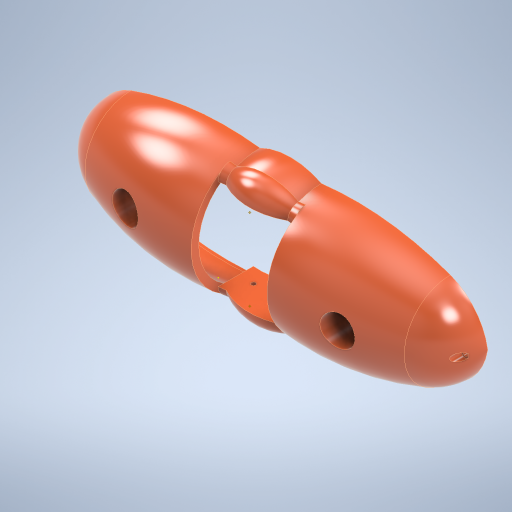
# Autodesk Inventor part: przód
Saved by Autodesk Inventor 2024 (Build 280153000, 153)
## iProperties
Created: 2025-05-21
Part Number: przód
Material: Tworzywo sztuczne PET
Document SubType Name: Modeling
Designer: Paweł
Density: 1.541 g/cm^3
Appearance: Gładki — jasnopomarańczowy
Mass: 215.204 g
Surface Area: 613.74 cm^2
Volume: 139.652 cm^3
Author: Paweł
Autodesk Inventor part; units mm, degrees
ref_plane "YZ Plane" through (0, 0, 0) normal (1, 0, 0) x (0, 1, 0)
sketch "Szkic1" plane through (0, 0, 0) normal (0, 0, 1) x (1, 0, 0)
  line L0 (19.3649, 0) -> (-19.3649, 0)
  line L1 (-19.3649, 0) -> (-103.6215, 0)
  line L2 (-103.6215, 0) -> (-125, 0)
  line L3 (-125, 0) -> (-103.6215, 0)
  line L4 (-103.6215, 0) -> (-19.3649, 0)
  line L5 (-19.3649, 0) -> (19.3649, 0)
  line L6 (19.3649, 0) -> (103.6215, 0)
  line L7 (103.6215, 0) -> (125, 0)
  line L8 (125, 0) -> (103.6215, 0)
  line L9 (103.6215, 0) -> (19.3649, 0)
  line L10 (45, 0) -> (-45, 0)
  line L11 (45, 0) -> (105.3748, 0)
  line L12 (105.3748, 0) -> (130.0712, 0)
  line L13 (130.0712, 0) -> (105.3748, 0)
  line L14 (105.3748, 0) -> (-20.2973, 0)
  line L15 (-20.2973, 0) -> (-105.3748, 0)
  line L16 (-105.3748, 0) -> (-105.3748, 0)
  line L17 (-105.3748, 0) -> (-130.0712, 0)
  line L18 (-130.0712, 0) -> (-105.3748, 0)
  line L19 (-105.3748, 0) -> (-45, 0)
  arc A0 (119.2902, -19.1594) -> (125, 0) centre (90, 0) ccw
  arc A1 (19.3649, -35) -> (103.6215, -25.7743) centre (42.8262, 140.0954) ccw
  arc A2 (103.6215, -25.7743) -> (125, 0) centre (91.4189, 6.1005) ccw
  arc A3 (20.2973, -40.1624) -> (105.3748, -30.457) centre (42.8262, 140.0954) ccw
  arc A4 (105.3748, -30.457) -> (130.0712, 0) centre (91.4189, 6.1005) ccw
  arc A5 (-125, 0) -> (-103.6215, -25.7743) centre (-91.4189, 6.1005) ccw
  arc A6 (-130.0712, 0) -> (-105.3748, -30.457) centre (-91.4189, 6.1005) ccw
  arc A7 (-98.4086, -33.9749) -> (-78.2644, -32.9739) centre (-90, 0) ccw
  arc A8 (-103.6215, -25.7743) -> (-19.3649, -35) centre (-42.8262, 140.0954) ccw
  arc A9 (-19.3649, -35) -> (19.3649, -35) centre (0, 0) ccw
  arc A10 (-20.2973, -40.1624) -> (20.2973, -40.1624) centre (0, 0) ccw
  arc A11 (-105.3748, -30.457) -> (-20.2973, -40.1624) centre (-42.8262, 140.0954) ccw
  line L20 (-105.3748, 0) -> (-20.2973, 0)
  line L21 (19.3649, 0) -> (-19.3649, 0)
  line L22 (130.0712, 0) -> (-130.0712, 0)
  point P0 (0, 0)
  point P1 (-119.2902, -19.1594)
  point P2 (-125, 0)
  point P3 (125, 0)
  dimension "d0" = 70
  dimension "d1" = 70
  dimension "d2" = 250
  dimension "d3" = 90
  constraints: 46 end point, 25 point on circle, 12 centre point, 2 horizontal alignment, 1 coincident, 1 horizontal, 4 other
  measures "d0" diameter of A0
  measures "d1" diameter of A7
  measures "d3" distance of point (0, 0) A7.centre
revolve "Obrót1" add sketch "Szkic1" angle 180 about axis through (130.0712, 0, 0) along (-1, 0, 0) contours L12 A4 A3 A10 A11 A7 A8 A9 A1 A2 | A5 A8 A7 A11 A6 L17
sketch "Szkic2" plane through (0, 0, 0) normal (0, 1, 0) x (-1, 0, 0)
  line L0 (-25, 45) -> (25, 45)
  line L1 (25, 45) -> (25, 15)
  line L2 (25, 15) -> (-25, 15)
  line L3 (-25, 15) -> (-25, 45)
  line L4 (-20.2973, 0) -> (20.2973, 0) projected
  arc A0 (105.3748, 30.457) -> (20.2973, 40.1624) centre (42.8262, -140.0954) ccw projected
  arc A1 (20.2973, 40.1624) -> (-20.2973, 40.1624) centre (0, 0) ccw projected
  point P0 (0, 0)
  point P1 (0, 45)
  point P2 (0, 0)
  point P3 (0, 45)
  dimension "d5" = 50
  dimension "d6" = 30
  constraints: 8 end point, 3 perpendicular, 2 midpoint, 1 coincident, 1 horizontal, 1 point on circle, 1 vertical alignment
  measures "d5" distance of L0.start L0.end
  measures "d6" distance of L0.end L1.end
extrude "Wyciągnięcie proste1" cut sketch "Szkic2" along normal mid plane 91
sketch "Szkic3" plane through (25, 0, 0) normal (-1, 0, 0) x (0, 0, 1)
  point P0 (0, 0)
sketch "Szkic11" plane through (0, 0, 15) normal (0, 0, 1) x (1, 0, 0)
  spline S0 degree 4 poles (25, -37.8222) (23.8224, -37.6973) (22.646, -37.5613) (21.4709, -37.4143) (20.2973, -37.2561) knots 0 0 0 0 0 1 1 1 1 1 projected
  line L0 (25, -32.3552) -> (25, -37.8222) projected
  spline S1 degree 7 poles (19.3649, -31.6228) (19.9801, -31.714) (20.5958, -31.8024) (21.2118, -31.888) (21.8282, -31.9707) (22.445, -32.0506) (23.0621, -32.1277) (23.8682, -32.2247) (24.0567, -32.2471) (24.2453, -32.2692) (24.4339, -32.2911) (24.6226, -32.3127) (24.8113, -32.3341) (25, -32.3552) knots 0 0 0 0 0 0 0 0 0.766096 0.766096 0.766096 0.766096 0.766096 0.766096 1 1 1 1 1 1 1 1 projected
  arc A0 (-19.3649, -31.6228) -> (19.3649, -31.6228) centre (0, 0) ccw projected
  spline S2 degree 4 poles (-25, -32.3552) (-23.5881, -32.1973) (-22.1781, -32.0227) (-20.7702, -31.8312) (-19.3649, -31.6228) knots 0 0 0 0 0 1 1 1 1 1 projected
  line L1 (-25, -37.8222) -> (-25, -32.3552) projected
  spline S3 degree 4 poles (-20.2973, -37.2561) (-21.4709, -37.4143) (-22.646, -37.5613) (-23.8224, -37.6973) (-25, -37.8222) knots 0 0 0 0 0 1 1 1 1 1 projected
  arc A1 (-20.2973, -37.2561) -> (20.2973, -37.2561) centre (0, 0) ccw projected
  line L2 (20, -30) -> (-20, -30) projected
  line L3 (-25, -30) -> (-20, -30) projected
  line L4 (-25, -32.3552) -> (-25, -30)
  line L5 (25, -32.3552) -> (25, -30)
  line L6 (25, -30) -> (20, -30)
  point P0 (0, 0)
  constraints: 6 end point, 2 perpendicular, 1 point on line, 4 other
revolve "Obrót2" add sketch "Szkic11" angle 105 about axis through (20, -30, 15) along (-1, 0, 0) contours S0 A1 S3 L1 S2 A0 S1 L0
sketch "Szkic12" plane through (0, 0, 15) normal (0, 0, 1) x (1, 0, 0)
  spline S0 degree 4 poles (20.2973, 37.2561) (21.4709, 37.4143) (22.646, 37.5613) (23.8224, 37.6973) (25, 37.8222) knots 0 0 0 0 0 1 1 1 1 1 projected
  arc A0 (20.2973, 37.2561) -> (-20.2973, 37.2561) centre (0, 0) ccw projected
  spline S1 degree 4 poles (-25, 37.8222) (-23.8224, 37.6973) (-22.646, 37.5613) (-21.4709, 37.4143) (-20.2973, 37.2561) knots 0 0 0 0 0 1 1 1 1 1 projected
  line L0 (-25, 32.3552) -> (-25, 37.8222) projected
  spline S2 degree 4 poles (-19.3649, 31.6228) (-20.7702, 31.8312) (-22.1781, 32.0227) (-23.5881, 32.1973) (-25, 32.3552) knots 0 0 0 0 0 1 1 1 1 1 projected
  arc A1 (19.3649, 31.6228) -> (-19.3649, 31.6228) centre (0, 0) ccw projected
  spline S3 degree 7 poles (25, 32.3552) (24.8113, 32.3341) (24.6226, 32.3127) (24.4339, 32.2911) (24.2453, 32.2692) (24.0567, 32.2471) (23.8682, 32.2247) (23.0621, 32.1277) (22.445, 32.0506) (21.8282, 31.9707) (21.2118, 31.888) (20.5958, 31.8024) (19.9801, 31.714) (19.3649, 31.6228) knots 0 0 0 0 0 0 0 0 0.233904 0.233904 0.233904 0.233904 0.233904 0.233904 1 1 1 1 1 1 1 1 projected
  line L1 (25, 37.8222) -> (25, 32.3552) projected
  line L2 (-20, 30) -> (20, 30) projected
  point P0 (0, 0)
  constraints: 4 other
revolve "Obrót3" add sketch "Szkic12" angle 105 about axis through (-20, 30, 15) along (1, 0, 0)
sketch "Szkic19" plane through (0, -37.7646, -13.9778) normal (0, 0.9659258, -0.258819) x (1, 0, 0)
  arc A0 (-19.3649, -31.6228) -> (19.3649, -31.6228) centre (0, 0) ccw projected
  ellipse E0 centre (-40.2575, 46.8732) end of major axis (73.1618, 50.4646) minor radius 80.1787 (-25, -32.3552) -> (-19.3649, -31.6228) ccw projected
  line L0 (-25, -32.3552) -> (-25, -37.1348) projected
  line L1 (-25, -37.8222) -> (-25, -37.1348) projected
  arc A1 (-25, -37.8222) -> (-20.2973, -37.2561) centre (-42.6902, 128.9635) ccw projected
  arc A2 (-20.2973, -37.2561) -> (20.2973, -37.2561) centre (0, 0) ccw projected
  arc A3 (20.2973, -37.2561) -> (25, -37.8222) centre (42.6902, 128.9635) ccw projected
  line L2 (25, -37.1348) -> (25, -37.8222) projected
  line L3 (25, -37.1348) -> (25, -32.3552) projected
  ellipse E1 centre (40.2575, 46.8732) end of major axis (153.6768, 43.2818) minor radius 80.1787 (19.3649, -31.6228) -> (25, -32.3552) ccw projected
  ellipse E2 centre (0, -23.2757) end of major axis (40, -23.2757) minor radius 10.3528 (19.3649, -14.217) -> (-19.3649, -14.217) ccw projected
  ellipse E3 centre (42.8262, -59.535) end of major axis (219.4864, -59.535) minor radius 45.723 (103.6215, -16.6048) -> (19.3649, -14.217) ccw projected
  ellipse E4 centre (-42.8262, -59.535) end of major axis (133.834, -59.535) minor radius 45.723 (-19.3649, -14.217) -> (-103.6215, -16.6048) ccw projected
  line L4 (-25, -32.3552) -> (-25, -14.0454)
  line L5 (25, -32.3552) -> (25, -14.0454)
  point P0 (0, -23.2757)
  constraints: 4 end point, 2 vertical, 7 other
extrude "Wyciągnięcie proste10" add sketch "Szkic19" against normal blind 6 contours E0 L4 E4 E2 E3 L5 E1 A0
sketch "Szkic20" plane through (0, 37.7646, -13.9778) normal (0, -0.9659258, -0.258819) x (1, 0, 0)
  arc A0 (-20.2973, 37.2561) -> (-25, 37.8222) centre (-42.6902, -128.9635) ccw projected
  line L0 (-25, 37.1348) -> (-25, 37.8222) projected
  line L1 (-25, 37.1348) -> (-25, 32.3552) projected
  ellipse E0 centre (-40.2575, -46.8732) end of major axis (73.1618, -50.4646) minor radius 80.1787 (-19.3649, 31.6228) -> (-25, 32.3552) ccw projected
  arc A1 (19.3649, 31.6228) -> (-19.3649, 31.6228) centre (0, 0) ccw projected
  ellipse E1 centre (40.2575, -46.8732) end of major axis (153.6768, -43.2818) minor radius 80.1787 (25, 32.3552) -> (19.3649, 31.6228) ccw projected
  line L2 (25, 32.3552) -> (25, 37.1348) projected
  line L3 (25, 37.8222) -> (25, 37.1348) projected
  arc A2 (25, 37.8222) -> (20.2973, 37.2561) centre (42.6902, -128.9635) ccw projected
  arc A3 (20.2973, 37.2561) -> (-20.2973, 37.2561) centre (0, 0) ccw projected
  ellipse E2 centre (42.8262, 59.535) end of major axis (219.4864, 59.535) minor radius 45.723 (19.3649, 14.217) -> (103.6215, 16.6048) ccw projected
  ellipse E3 centre (0, 23.2757) end of major axis (40, 23.2757) minor radius 10.3528 (-19.3649, 14.217) -> (19.3649, 14.217) ccw projected
  ellipse E4 centre (-42.8262, 59.535) end of major axis (133.834, 59.535) minor radius 45.723 (-103.6215, 16.6048) -> (-19.3649, 14.217) ccw projected
  line L4 (-25, 32.3552) -> (-25, 14.0454)
  line L5 (25, 32.3552) -> (25, 14.0454)
  point P0 (0, 23.2757)
  constraints: 4 end point, 2 vertical, 7 other
extrude "Wyciągnięcie proste11" add sketch "Szkic20" against normal blind 6 contours E0 A1 E1 L5 E2 E3 E4 L4
ref_plane "Płaszczyzna konstrukcyjna2" through (0, 26.7838, 27.003) normal (0, 1, 0) x (-1, 0, 0)
sketch "Szkic22" plane through (0, 26.7838, 27.003) normal (0, 1, 0) x (-1, 0, 0)
  ellipse E0 centre (42.6902, -165.5499) end of major axis (210.4114, -165.5499) minor radius 162.0063 (25, -4.4473) -> (20.2973, -4.9941) ccw projected
  line L0 (25, -5.1113) -> (25, -4.4473) projected
  line L1 (25, -5.1113) -> (25, -27.414) projected
  ellipse E1 centre (42.8262, 16.5257) end of major axis (-133.834, 16.5257) minor radius 44.1651 (19.3649, -27.2482) -> (25, -27.414) ccw projected
  ellipse E2 centre (0, -18.4982) end of major axis (-40, -18.4982) minor radius 10 (-19.3649, -27.2482) -> (19.3649, -27.2482) ccw projected
  ellipse E3 centre (-42.8262, 16.5257) end of major axis (-219.4864, 16.5257) minor radius 44.1651 (-25, -27.414) -> (-19.3649, -27.2482) ccw projected
  line L2 (-25, -27.414) -> (-25, -5.1113) projected
  line L3 (-25, -4.4473) -> (-25, -5.1113) projected
  ellipse E4 centre (-42.6902, -165.5499) end of major axis (125.031, -165.5499) minor radius 162.0063 (-20.2973, -4.9941) -> (-25, -4.4473) ccw projected
  ellipse E5 centre (0, -40.9808) end of major axis (42.4264, -40.9808) minor radius 40.9808 (20.2973, -4.9941) -> (-20.2973, -4.9941) ccw projected
  point P0 (0, -27.003)
  constraints: 6 other
extrude "Wyciągnięcie proste12" add sketch "Szkic22" along normal up to surface surface through (0, 28.1821, 21.7846) normal (0, -0.9659258, -0.258819)
ref_plane "Płaszczyzna konstrukcyjna3" through (0, -26.7838, 27.003) normal (0, 1, 0) x (-1, 0, 0)
sketch "Szkic23" plane through (0, -26.7838, 27.003) normal (0, 1, 0) x (-1, 0, 0)
  line L0 (25, -27.414) -> (25, -5.1113) projected
  line L1 (25, -4.4473) -> (25, -5.1113) projected
  ellipse E0 centre (42.6902, -165.5499) end of major axis (-125.031, -165.5499) minor radius 162.0063 (25, -4.4473) -> (20.2973, -4.9941) ccw projected
  ellipse E1 centre (0, -40.9808) end of major axis (-42.4264, -40.9808) minor radius 40.9808 (20.2973, -4.9941) -> (-20.2973, -4.9941) ccw projected
  ellipse E2 centre (-42.6902, -165.5499) end of major axis (-210.4114, -165.5499) minor radius 162.0063 (-20.2973, -4.9941) -> (-25, -4.4473) ccw projected
  line L2 (-25, -5.1113) -> (-25, -4.4473) projected
  line L3 (-25, -5.1113) -> (-25, -27.414) projected
  ellipse E3 centre (-42.8262, 16.5257) end of major axis (-219.4864, 16.5257) minor radius 44.1651 (-25, -27.414) -> (-19.3649, -27.2482) ccw projected
  ellipse E4 centre (0, -18.4982) end of major axis (-40, -18.4982) minor radius 10 (-19.3649, -27.2482) -> (19.3649, -27.2482) ccw projected
  ellipse E5 centre (42.8262, 16.5257) end of major axis (-133.834, 16.5257) minor radius 44.1651 (19.3649, -27.2482) -> (25, -27.414) ccw projected
  point P0 (0, -27.003)
  constraints: 6 other
extrude "Wyciągnięcie proste13" add sketch "Szkic23" against normal up to surface surface through (0, -28.1821, 21.7846) normal (0, 0.9659258, -0.258819)
sketch "Szkic24" plane through (0, 0, 0) normal (0, 0, -1) x (-1, 0, 0)
  line L0 (-32.3004, 30) -> (-32.3004, -30)
  line L1 (-32.3004, -30) -> (32.3004, -30)
  line L2 (20.2973, -37.2561) -> (20.2973, -28.122) projected
  line L3 (32.3004, -30) -> (32.3004, 30)
  line L4 (32.3004, 30) -> (-32.3004, 30)
  line L5 (-25, -27.6243) -> (-25, 27.6243) projected
  line L6 (25, 27.6243) -> (25, -27.6243) projected
  line L7 (25, 26.7838) -> (25, 34.1294) projected
  line L8 (25, -26.7838) -> (25, -34.1294) projected
  line L9 (-25, -26.7838) -> (-25, -34.1294) projected
  line L10 (-25, 26.7838) -> (-25, 34.1294) projected
  point P0 (0, 0)
  point P1 (-32.3004, 0)
  point P2 (0, -30)
  point P3 (-25, 30)
  point P4 (-25, -30)
  point P5 (25, -30)
  point P6 (25, 30)
  dimension "d41" = 60
  constraints: 8 end point, 3 perpendicular, 2 midpoint, 1 horizontal alignment, 1 vertical, 1 vertical alignment
  measures "d41" distance of L0.start L0.end
extrude "Wyciągnięcie proste14" cut sketch "Szkic24" along normal blind 10 and the other way blind 49 contours L4 L7 L6 L8 L1 L9 L5 L10
sketch "Szkic25" plane through (0, -30, -15) normal (0, 1, 0) x (1, 0, 0)
  circle A0 centre (15, -24.589) radius 1.5
  circle A1 centre (-15, -24.589) radius 1.5
  line L0 (25, -14.589) -> (25, -34.2836) projected
  point P0 (0, -15)
  dimension "d46" = 3
  dimension "d47" = 3
  dimension "d48" = 30
  dimension "d49" = 10
  dimension "d50" = 10
  dimension "d67" = 10
  constraints: 2 centre point
  measures "d46" diameter of A0
  measures "d47" diameter of A1
  measures "d48" distance of A0.centre A1.centre
  measures "d49" distance from line of A0.centre L0
  measures "d50" horizontal distance of A0.centre L0.start
  measures "d67" vertical distance of L0.start A1.centre
extrude "Wyciągnięcie proste15" cut sketch "Szkic25" against normal blind 10
sketch "Szkic26" plane through (0, 0, 0) normal (0, 0, 1) x (1, 0, 0)
  circle A0 centre (-70, 0) radius 10
  circle A1 centre (70, 0) radius 10
  circle A2 centre (-70, 0) radius 12
  circle A3 centre (70, 0) radius 12
  point P0 (0, 0)
  dimension "d53" = 20
  dimension "d54" = 20
  dimension "d55" = 70
  dimension "d56" = 70
  dimension "d59" = 2
  dimension "d60" = 2
  constraints: 4 centre point, 2 horizontal alignment
  measures "d53" diameter of A0
  measures "d54" diameter of A1
  measures "d55" distance of A1.centre point (0, 0)
  measures "d56" distance of A0.centre point (0, 0)
  measures "d59" radial gap between concentric circles of A0 A2
  measures "d60" radial gap between concentric circles of A1 A3
extrude "Wyciągnięcie proste16" cut sketch "Szkic26" along normal blind 50 contours A0 | A1
extrude "Wyciągnięcie proste17" add sketch "Szkic26" along normal up to surface contours A2
extrude "Wyciągnięcie proste18" add sketch "Szkic26" along normal up to surface contours A3
extrude "Wyciągnięcie proste19" cut sketch "Szkic26" along normal blind 23 contours A0 | A2 | A3
sketch "Szkic28" plane through (0, 0, 0) normal (0, 0, -1) x (-1, 0, 0)
  arc A0 (105.3748, -30.457) -> (130.0712, 0) centre (91.4189, 6.1005) ccw projected
  arc A1 (130.0712, 0) -> (105.3748, 30.457) centre (91.4189, -6.1005) ccw projected
  circle A2 centre (125, 0) radius 5
  circle A3 centre (125, 0) radius 2.5
  line L0 (0, 0) -> (0, 11.9782)
  arc A4 (-130.0712, 0) -> (-105.3748, -30.457) centre (-91.4189, 6.1005) ccw
  arc A5 (-105.3748, 30.457) -> (-130.0712, 0) centre (-91.4189, -6.1005) ccw
  circle A6 centre (-125, 0) radius 5
  circle A7 centre (-125, 0) radius 2.5
  dimension "d79" = 10
  dimension "d85" = 5
  constraints: 7 symmetric about line, 6 centre point, 4 point on circle, 2 coincident, 2 end point, 2 tangent, 1 vertical, 4 other
  measures "d79" diameter of A2
  measures "d85" diameter of A3
extrude "Wyciągnięcie proste21" add sketch "Szkic28" against normal blind 8.5 contours A3 | A7
ref_plane "Płaszczyzna konstrukcyjna4" through (0, 0, 47.75) normal (0, 0, -1) x (-1, 0, 0)
sketch "Szkic34" plane through (0, 0, 47.75) normal (0, 0, -1) x (-1, 0, 0)
  point P0 (0, 0)
sketch "Szkic35" plane through (0, 0, 47.75) normal (0, 0, -1) x (-1, 0, 0)
  arc A0 (124.4634, 2.4417) -> (124.4634, -2.4417) centre (125, 0) ccw projected
  circle A1 centre (125, 0) radius 2.5
  line L0 (0, 0) -> (0, -27.9638)
  arc A2 (-124.4634, -2.4417) -> (-124.4634, 2.4417) centre (-125, 0) ccw
  circle A3 centre (-125, 0) radius 2.5
  point P0 (124.4634, -2.4417)
  point P1 (124.4634, 2.4417)
  point P2 (-124.4634, 2.4417)
  point P3 (-124.4634, -2.4417)
  constraints: 4 symmetric about line, 3 centre point, 2 coincident, 2 end point, 2 point on circle, 1 vertical, 2 other
extrude "Wyciągnięcie proste26" cut sketch "Szkic35" along normal blind 38
sketch "Szkic36" plane through (0, 0, 9.75) normal (0, 0, 1) x (1, 0, 0)
  arc A0 (-127.1597, -1.2593) -> (-127.1597, 1.2593) centre (-125, 0) ccw projected
  circle A1 centre (-125, 0) radius 1.5
  line L0 (0, 0) -> (0, -13.6342)
  circle A2 centre (125, 0) radius 1.5
  dimension "d89" = 3
  constraints: 2 centre point, 2 end point, 1 coincident, 1 symmetric about line, 1 vertical, 1 other
  measures "d89" diameter of A1
extrude "Wyciągnięcie proste27" cut sketch "Szkic36" against normal blind 38
sketch "Szkic37" plane through (0, 0, 0) normal (0, 0, -1) x (-1, 0, 0)
  point P0 (0, 0)
sketch "Szkic38" plane through (0, 0, 0) normal (0, 0, -1) x (-1, 0, 0)
  arc A0 (-127.1597, -1.2593) -> (-127.1597, 1.2593) centre (-125, 0) ccw projected
  circle A1 centre (-125, 0) radius 5
  circle A2 centre (125, 0) radius 1.5 projected
  circle A3 centre (125, 0) radius 5
  arc A4 (-124.4634, -2.4417) -> (-103.6215, -25.7743) centre (-91.4189, 6.1005) ccw projected
  arc A5 (-103.6215, 25.7743) -> (-124.4634, 2.4417) centre (-91.4189, -6.1005) ccw projected
  point P0 (0, 0)
  point P1 (-123.7484, 4.8408)
  point P2 (-123.7484, -4.8408)
  dimension "d92" = 10
  dimension "d93" = 10
  constraints: 2 centre point, 2 coincident
  measures "d92" diameter of A1
  measures "d93" diameter of A3
extrude "Wyciągnięcie proste28" add sketch "Szkic38" against normal up to surface contours A0 A5 A1 A4 picked at (-122.8056, -3.5127)
sketch "Szkic39" plane through (0, 0, 0) normal (0, 0, -1) x (-1, 0, 0)
  circle A0 centre (125, 0) radius 1.5 projected
  circle A1 centre (125, 0) radius 5
  arc A2 (103.6215, -25.7743) -> (124.4634, -2.4417) centre (91.4189, 6.1005) ccw projected
  arc A3 (124.4634, 2.4417) -> (103.6215, 25.7743) centre (91.4189, -6.1005) ccw projected
  arc A4 (124.4634, 2.4417) -> (124.4634, -2.4417) centre (125, 0) ccw projected
  point P0 (0, 0)
  point P1 (123.7484, 4.8408)
  point P2 (123.7484, -4.8408)
  dimension "d96" = 10
  constraints: 1 centre point, 1 coincident
  measures "d96" diameter of A1
extrude "Wyciągnięcie proste29" add sketch "Szkic39" against normal up to surface contours A3 A4 A2 A1 picked at (120.8635, 0.1024)
sketch "Szkic40" plane through (0, 0, 0) normal (0, 0, -1) x (-1, 0, 0)
  arc A0 (103.6215, -25.7743) -> (123.7484, -4.8408) centre (91.4189, 6.1005) ccw projected
  arc A1 (25, -35.6631) -> (103.6215, -25.7743) centre (42.8262, 140.0954) ccw projected
  arc A2 (19.3649, -35) -> (25, -35.6631) centre (42.8262, 140.0954) ccw projected
  arc A3 (-19.3649, -35) -> (19.3649, -35) centre (0, 0) ccw projected
  arc A4 (-25, -35.6631) -> (-19.3649, -35) centre (-42.8262, 140.0954) ccw projected
  arc A5 (-103.6215, -25.7743) -> (-25, -35.6631) centre (-42.8262, 140.0954) ccw projected
  arc A6 (-123.7484, -4.8408) -> (-103.6215, -25.7743) centre (-91.4189, 6.1005) ccw projected
  arc A7 (-123.7484, -4.8408) -> (-123.7484, 4.8408) centre (-125, 0) ccw projected
  arc A8 (-103.6215, 25.7743) -> (-123.7484, 4.8408) centre (-91.4189, -6.1005) ccw projected
  arc A9 (-25, 35.6631) -> (-103.6215, 25.7743) centre (-42.8262, -140.0954) ccw projected
  arc A10 (-19.3649, 35) -> (-25, 35.6631) centre (-42.8262, -140.0954) ccw projected
  arc A11 (19.3649, 35) -> (-19.3649, 35) centre (0, 0) ccw projected
  arc A12 (25, 35.6631) -> (19.3649, 35) centre (42.8262, -140.0954) ccw projected
  arc A13 (103.6215, 25.7743) -> (25, 35.6631) centre (42.8262, -140.0954) ccw projected
  arc A14 (123.7484, 4.8408) -> (103.6215, 25.7743) centre (91.4189, -6.1005) ccw projected
  arc A15 (123.7484, 4.8408) -> (123.7484, -4.8408) centre (125, 0) ccw projected
  circle A16 centre (125, 0) radius 1.5 projected
  circle A17 centre (-125, 0) radius 1.5 projected
  arc A18 (-130.0712, 0) -> (-105.3748, -30.457) centre (-91.4189, 6.1005) ccw projected
  arc A19 (-105.3748, -30.457) -> (-20.2973, -40.1624) centre (-42.8262, 140.0954) ccw projected
  arc A20 (-20.2973, -40.1624) -> (20.2973, -40.1624) centre (0, 0) ccw projected
  arc A21 (20.2973, -40.1624) -> (105.3748, -30.457) centre (42.8262, 140.0954) ccw projected
  arc A22 (105.3748, -30.457) -> (130.0712, 0) centre (91.4189, 6.1005) ccw projected
  arc A23 (130.0712, 0) -> (105.3748, 30.457) centre (91.4189, -6.1005) ccw projected
  arc A24 (105.3748, 30.457) -> (20.2973, 40.1624) centre (42.8262, -140.0954) ccw projected
  arc A25 (20.2973, 40.1624) -> (-20.2973, 40.1624) centre (0, 0) ccw projected
  arc A26 (-20.2973, 40.1624) -> (-105.3748, 30.457) centre (-42.8262, -140.0954) ccw projected
  arc A27 (-105.3748, 30.457) -> (-130.0712, 0) centre (-91.4189, -6.1005) ccw projected
  arc A28 (-104.323, 27.6473) -> (-126.4847, 2.6068) centre (-91.4189, -6.1005) ccw
  arc A29 (-126.4847, -2.6068) -> (-126.4847, 2.6068) centre (-125, 0) ccw
  arc A30 (-126.4847, -2.6068) -> (-104.323, -27.6473) centre (-91.4189, 6.1005) ccw
  arc A31 (-104.323, -27.6473) -> (-24.7982, -37.6529) centre (-42.8262, 140.0954) ccw
  arc A32 (-24.7982, -37.6529) -> (-19.7476, -37.0679) centre (-42.8262, 140.0954) ccw
  arc A33 (-19.7476, -37.0679) -> (19.7476, -37.0679) centre (0, 0) ccw
  arc A34 (19.7476, -37.0679) -> (24.7982, -37.6529) centre (42.8262, 140.0954) ccw
  arc A35 (24.7982, -37.6529) -> (104.323, -27.6473) centre (42.8262, 140.0954) ccw
  arc A36 (104.323, -27.6473) -> (126.4847, -2.6068) centre (91.4189, 6.1005) ccw
  arc A37 (126.4847, 2.6068) -> (126.4847, -2.6068) centre (125, 0) ccw
  arc A38 (126.4847, 2.6068) -> (104.323, 27.6473) centre (91.4189, -6.1005) ccw
  arc A39 (104.323, 27.6473) -> (24.7982, 37.6529) centre (42.8262, -140.0954) ccw
  arc A40 (24.7982, 37.6529) -> (19.7476, 37.0679) centre (42.8262, -140.0954) ccw
  arc A41 (19.7476, 37.0679) -> (-19.7476, 37.0679) centre (0, 0) ccw
  arc A42 (-19.7476, 37.0679) -> (-24.7982, 37.6529) centre (-42.8262, -140.0954) ccw
  arc A43 (-24.7982, 37.6529) -> (-104.323, 27.6473) centre (-42.8262, -140.0954) ccw
  arc A44 (126.4847, -2.6068) -> (127.0309, 0) centre (91.4189, 6.1005) ccw
  arc A45 (127.0309, 0) -> (126.4847, 2.6068) centre (91.4189, -6.1005) ccw
  arc A46 (-127.0309, 0) -> (-126.4847, -2.6068) centre (-91.4189, 6.1005) ccw
  arc A47 (-126.4847, 2.6068) -> (-127.0309, 0) centre (-91.4189, -6.1005) ccw
  point P0 (0, 0)
  dimension "d99" = 2
  constraints: 40 point on circle, 20 centre point, 15 other
  measures "d99" radial gap between concentric circles of A9 A43
extrude "Wyciągnięcie proste30" add sketch "Szkic40" along normal blind 2 contours A43 A42 A41 A40 A39 A38 A37 A36 A35 A34 A33 A32 A31 A30 A29 A28 | A29 A46 A47 | A45 A44 A37
equation "\"d57\" = d5"
equation "\"d61\" = d5"
